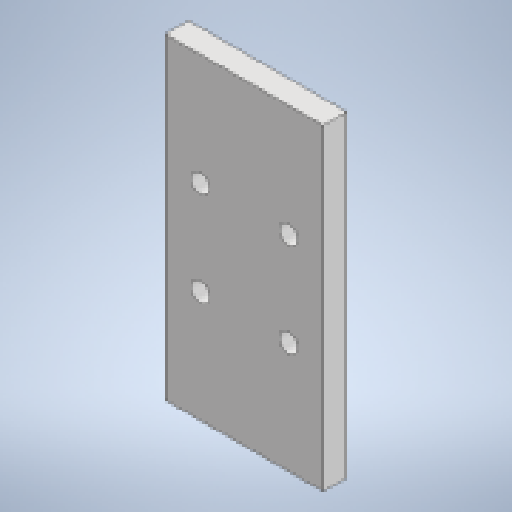
# Autodesk Inventor part: фанера_креп_маркера
Saved by Autodesk Inventor 2023.1 (Build 271208000, 208)
## iProperties
Created: 2026-01-10
Part Number: фанера_креп_маркера
Material: Типовые
Document SubType Name: Modeling
Designer: DELL
Density: 1 g/cm^3
Appearance: По умолчанию
Author: DELL
Autodesk Inventor part; units mm, degrees
ref_plane "YZ Plane" through (0, 0, 0) normal (1, 0, 0) x (0, 1, 0)
ref_plane "XZ Plane" through (0, 0, 0) normal (0, 1, 0) x (-1, 0, 0)
ref_plane "XY Plane" through (0, 0, 0) normal (0, 0, 1) x (1, 0, 0)
sketch "Эскиз1" plane through (0, 0, 0) normal (0, 0, 1) x (1, 0, 0)
  line L0 (-13.5, -49) -> (13.5, -49) projected
  line L1 (13.5, -49) -> (13.5, 5) projected
  line L2 (13.5, 5) -> (-13.5, 5) projected
  line L3 (-13.5, 5) -> (-13.5, -49) projected
  circle A0 centre (-7.5, -30) radius 1.6 projected
  circle A1 centre (7.5, -30) radius 1.6 projected
  circle A2 centre (7.5, -14) radius 1.6 projected
  circle A3 centre (-7.5, -14) radius 1.6 projected
  point P0 (0, 0)
extrude "Выдавливание1" add sketch "Эскиз1" along normal blind 4
